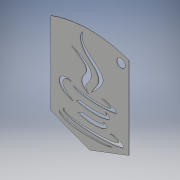
# Autodesk Inventor part: Деталь1
Saved by Autodesk Inventor 2018 (Build 220112000, 112)
## iProperties
Created: 2019-05-28
Part Number: Деталь1
Material: Типовые
Document SubType Name: Modeling
Designer: Vdalilsav
Density: 1 g/cm^3
Appearance: По умолчанию
Author: Vdalilsav
Autodesk Inventor part; units mm, degrees
ref_plane "YZ Plane" through (0, 0, 0) normal (1, 0, 0) x (0, 1, 0)
ref_plane "XZ Plane" through (0, 0, 0) normal (0, 1, 0) x (-1, 0, 0)
ref_plane "XY Plane" through (0, 0, 0) normal (0, 0, 1) x (1, 0, 0)
sketch "Эскиз1" plane through (0, 0, 0) normal (0, 1, 0) x (-1, 0, 0)
  line L0 (-168.2014, 197.6883) -> (149.2986, 197.6883) construction
  line L1 (149.2986, 197.6883) -> (149.2986, -384.3951) construction
  line L2 (149.2986, -384.3951) -> (-168.2014, -384.3951) construction
  line L3 (-168.2014, -384.3951) -> (-168.2014, 197.6883) construction
  line L4 (-172.8134, 183.0403) -> (-172.8134, -183.0403)
  line L5 (172.8134, -183.0403) -> (172.8134, 183.0403)
  line L6 (172.8134, 183.0403) -> (-172.8134, -183.0403) construction
  line L7 (-172.8134, 183.0403) -> (172.8134, -183.0403) construction
  line L8 (172.8134, -183.0403) -> (0, -248.8926)
  line L9 (-172.8134, -183.0403) -> (0, -248.8926)
  arc A0 (172.8134, 183.0403) -> (-172.8134, 183.0403) centre (0, -289.2463) ccw
  point P0 (0, 0)
  constraints: 12 end point, 2 midpoint, 2 point on circle, 1 centre point, 1 parallel, 2 other
sketch "Эскиз2" plane through (0, 0, 0) normal (0, 1, 0) x (-1, 0, 0)
  line L0 (-100.5732, -187.6969) -> (-90.8844, -191.9808) construction
  line L1 (-90.8844, -191.9808) -> (-75.4303, -195.3039) construction
  line L2 (-75.4303, -195.3039) -> (-57.8073, -197.5462) construction
  line L3 (-57.8073, -197.5462) -> (-50.4484, -198.1122) construction
  line L4 (-50.4484, -198.1122) -> (11.3731, -199.5671) construction
  line L5 (11.3731, -199.5671) -> (22.1637, -199.159) construction
  line L6 (22.1637, -199.159) -> (72.6522, -194.6635) construction
  line L7 (72.6522, -194.6635) -> (84.5907, -192.6655) construction
  line L8 (84.5907, -192.6655) -> (101.2161, -188.5411) construction
  line L9 (101.2161, -188.5411) -> (113.2372, -184.745) construction
  line L10 (113.2372, -184.745) -> (121.2017, -180.7255) construction
  line L11 (121.2017, -180.7255) -> (127.9007, -176.5944) construction
  line L12 (127.9007, -176.5944) -> (132.2272, -172.7909) construction
  line L13 (132.2272, -172.7909) -> (135.5715, -167.456) construction
  line L14 (135.5715, -167.456) -> (136.6862, -164.271) construction
  line L15 (136.6862, -164.271) -> (136.8189, -162.6519) construction
  line L16 (136.8189, -162.6519) -> (135.253, -164.271) construction
  line L17 (135.253, -164.271) -> (131.9353, -167.1375) construction
  line L18 (131.9353, -167.1375) -> (128.5645, -169.4201) construction
  line L19 (128.5645, -169.4201) -> (123.3836, -172.1896) construction
  line L20 (123.3836, -172.1896) -> (115.4536, -175.3114) construction
  line L21 (115.4536, -175.3114) -> (105.0835, -178.6485) construction
  line L22 (105.0835, -178.6485) -> (97.8352, -180.7655) construction
  line L23 (97.8352, -180.7655) -> (89.5822, -182.8826) construction
  line L24 (89.5822, -182.8826) -> (69.3615, -186.6907) construction
  line L25 (69.3615, -186.6907) -> (41.7588, -190.329) construction
  line L26 (41.7588, -190.329) -> (25.8958, -191.6874) construction
  line L27 (25.8958, -191.6874) -> (13.6226, -192.4635) construction
  line L28 (13.6226, -192.4635) -> (-0.2444, -193.1249) construction
  line L29 (-0.2444, -193.1249) -> (-15.9321, -193.513) construction
  line L30 (-15.9321, -193.513) -> (-21.243, -193.3904) construction
  line L31 (-21.243, -193.3904) -> (-33.8836, -193.3904) construction
  line L32 (-33.8836, -193.3904) -> (-40.4709, -193.2688) construction
  line L33 (-40.4709, -193.2688) -> (-51.2014, -192.7429) construction
  line L34 (-51.2014, -192.7429) -> (-59.6148, -192.1507) construction
  line L35 (-59.6148, -192.1507) -> (-65.0181, -191.7806) construction
  line L36 (-65.0181, -191.7806) -> (-74.3451, -191.0632) construction
  line L37 (-74.3451, -191.0632) -> (-76.1112, -190.9177) construction
  line L38 (-76.1112, -190.9177) -> (-91.5755, -189.204) construction
  line L39 (-91.5755, -189.204) -> (-94.5965, -188.6807) construction
  line L40 (-94.5965, -188.6807) -> (-97.0229, -188.3952) construction
  line L41 (-97.0229, -188.3952) -> (-98.5454, -188.1335) construction
  line L42 (-98.5454, -188.1335) -> (-100.5732, -187.6969) construction
  spline S0 degree 4 poles (-100.5732, -187.6969) (-90.8844, -191.9808) (-75.4303, -195.3039) (-57.8073, -197.5462) (-50.4484, -198.1122) (11.3731, -199.5671) (22.1637, -199.159) (72.6522, -194.6635) (84.5907, -192.6655) (101.2161, -188.5411) (113.2372, -184.745) (121.2017, -180.7255) (127.9007, -176.5944) (132.2272, -172.7909) (135.5715, -167.456) (136.6862, -164.271) (136.8189, -162.6519) (135.253, -164.271) (131.9353, -167.1375) (128.5645, -169.4201) (123.3836, -172.1896) (115.4536, -175.3114) (105.0835, -178.6485) (97.8352, -180.7655) (89.5822, -182.8826) (69.3615, -186.6907) (41.7588, -190.329) (25.8958, -191.6874) (13.6226, -192.4635) (-0.2444, -193.1249) (-15.9321, -193.513) (-21.243, -193.3904) (-33.8836, -193.3904) (-40.4709, -193.2688) (-51.2014, -192.7429) (-59.6148, -192.1507) (-65.0181, -191.7806) (-74.3451, -191.0632) (-76.1112, -190.9177) (-91.5755, -189.204) (-94.5965, -188.6807) (-97.0229, -188.3952) (-98.5454, -188.1335) (-100.5732, -187.6969) knots 1 1 1 1 1 2 3 4 5 6 7 8 9 10 11 12 13 14 15 16 17 18 19 20 21 22 23 24 25 26 27 28 29 30 31 32 33 34 35 36 37 38 39 40 41 41 41 41 41
  line L43 (111.9403, -142.3432) -> (113.6459, -144.4752) construction
  line L44 (113.6459, -144.4752) -> (114.6054, -147.6732) construction
  line L45 (114.6054, -147.6732) -> (113.7952, -150.1677) construction
  line L46 (113.7952, -150.1677) -> (110.892, -153.4059) construction
  line L47 (110.892, -153.4059) -> (108.3804, -154.9455) construction
  line L48 (108.3804, -154.9455) -> (102.2402, -157.513) construction
  line L49 (102.2402, -157.513) -> (97.2683, -159.1703) construction
  line L50 (97.2683, -159.1703) -> (86.7866, -161.5025) construction
  line L51 (86.7866, -161.5025) -> (78.9079, -162.7514) construction
  line L52 (78.9079, -162.7514) -> (72.2047, -164.0736) construction
  line L53 (72.2047, -164.0736) -> (49.1932, -166.8955) construction
  line L54 (49.1932, -166.8955) -> (37.3998, -167.7645) construction
  line L55 (37.3998, -167.7645) -> (18.7176, -169.2206) construction
  line L56 (18.7176, -169.2206) -> (-3.2892, -169.9456) construction
  line L57 (-3.2892, -169.9456) -> (-37.5273, -169.9456) construction
  line L58 (-37.5273, -169.9456) -> (-70.3936, -168.8122) construction
  line L59 (-70.3936, -168.8122) -> (-96.3775, -166.0991) construction
  line L60 (-96.3775, -166.0991) -> (-107.3306, -164.11) construction
  line L61 (-107.3306, -164.11) -> (-118.6934, -161.143) construction
  line L62 (-118.6934, -161.143) -> (-125.7296, -158.4458) construction
  line L63 (-125.7296, -158.4458) -> (-127.6116, -155.8998) construction
  line L64 (-127.6116, -155.8998) -> (-127.6116, -154.0071) construction
  line L65 (-127.6116, -154.0071) -> (-122.7322, -149.8816) construction
  line L66 (-122.7322, -149.8816) -> (-119.7589, -148.3776) construction
  line L67 (-119.7589, -148.3776) -> (-107.9616, -143.9347) construction
  line L68 (-107.9616, -143.9347) -> (-99.7456, -142.3432) construction
  line L69 (-99.7456, -142.3432) -> (-94.4887, -141.5856) construction
  line L70 (-94.4887, -141.5856) -> (-90.6183, -141.5856) construction
  line L71 (-90.6183, -141.5856) -> (-89.6238, -141.1555) construction
  line L72 (-89.6238, -141.1555) -> (-92.4191, -139.9192) construction
  line L73 (-92.4191, -139.9192) -> (-100.3212, -138.9516) construction
  line L74 (-100.3212, -138.9516) -> (-106.2881, -139.3547) construction
  line L75 (-106.2881, -139.3547) -> (-117.309, -141.3671) construction
  line L76 (-117.309, -141.3671) -> (-124.6465, -143.4482) construction
  line L77 (-124.6465, -143.4482) -> (-132.0085, -146.0648) construction
  line L78 (-132.0085, -146.0648) -> (-139.1832, -149.2139) construction
  line L79 (-139.1832, -149.2139) -> (-146.6729, -153.6575) construction
  line L80 (-146.6729, -153.6575) -> (-151.7202, -158.4964) construction
  line L81 (-151.7202, -158.4964) -> (-152.3684, -159.7625) construction
  line L82 (-152.3684, -159.7625) -> (-152.744, -162.9865) construction
  line L83 (-152.744, -162.9865) -> (-150.9599, -166.2105) construction
  line L84 (-150.9599, -166.2105) -> (-145.5761, -169.0589) construction
  line L85 (-145.5761, -169.0589) -> (-119.9974, -174.2608) construction
  line L86 (-119.9974, -174.2608) -> (-101.9283, -176.7574) construction
  line L87 (-101.9283, -176.7574) -> (-87.3291, -178.2385) construction
  line L88 (-87.3291, -178.2385) -> (-48.1035, -180.7168) construction
  line L89 (-48.1035, -180.7168) -> (-31.7211, -180.7168) construction
  line L90 (-31.7211, -180.7168) -> (22.8506, -178.8966) construction
  line L91 (22.8506, -178.8966) -> (35.2716, -177.6179) construction
  line L92 (35.2716, -177.6179) -> (61.13, -174.1701) construction
  line L93 (61.13, -174.1701) -> (82.266, -169.9038) construction
  line L94 (82.266, -169.9038) -> (93.8598, -166.6471) construction
  line L95 (93.8598, -166.6471) -> (105.7687, -161.9975) construction
  line L96 (105.7687, -161.9975) -> (113.4351, -158.2051) construction
  line L97 (113.4351, -158.2051) -> (118.7211, -153.0885) construction
  line L98 (118.7211, -153.0885) -> (119.8393, -149.2257) construction
  line L99 (119.8393, -149.2257) -> (118.6194, -146.8538) construction
  line L100 (118.6194, -146.8538) -> (116.4169, -144.8207) construction
  line L101 (116.4169, -144.8207) -> (112.6896, -142.6182) construction
  line L102 (112.6896, -142.6182) -> (111.9403, -142.3432) construction
  spline S1 degree 4 poles (111.9403, -142.3432) (113.6459, -144.4752) (114.6054, -147.6732) (113.7952, -150.1677) (110.892, -153.4059) (108.3804, -154.9455) (102.2402, -157.513) (97.2683, -159.1703) (86.7866, -161.5025) (78.9079, -162.7514) (72.2047, -164.0736) (49.1932, -166.8955) (37.3998, -167.7645) (18.7176, -169.2206) (-3.2892, -169.9456) (-37.5273, -169.9456) (-70.3936, -168.8122) (-96.3775, -166.0991) (-107.3306, -164.11) (-118.6934, -161.143) (-125.7296, -158.4458) (-127.6116, -155.8998) (-127.6116, -154.0071) (-122.7322, -149.8816) (-119.7589, -148.3776) (-107.9616, -143.9347) (-99.7456, -142.3432) (-94.4887, -141.5856) (-90.6183, -141.5856) (-89.6238, -141.1555) (-92.4191, -139.9192) (-100.3212, -138.9516) (-106.2881, -139.3547) (-117.309, -141.3671) (-124.6465, -143.4482) (-132.0085, -146.0648) (-139.1832, -149.2139) (-146.6729, -153.6575) (-151.7202, -158.4964) (-152.3684, -159.7625) (-152.744, -162.9865) (-150.9599, -166.2105) (-145.5761, -169.0589) (-119.9974, -174.2608) (-101.9283, -176.7574) (-87.3291, -178.2385) (-48.1035, -180.7168) (-31.7211, -180.7168) (22.8506, -178.8966) (35.2716, -177.6179) (61.13, -174.1701) (82.266, -169.9038) (93.8598, -166.6471) (105.7687, -161.9975) (113.4351, -158.2051) (118.7211, -153.0885) (119.8393, -149.2257) (118.6194, -146.8538) (116.4169, -144.8207) (112.6896, -142.6182) (111.9403, -142.3432) knots 1 1 1 1 1 2 3 4 5 6 7 8 9 10 11 12 13 14 15 16 17 18 19 20 21 22 23 24 25 26 27 28 29 30 31 32 33 34 35 36 37 38 39 40 41 42 43 44 45 46 47 48 49 50 51 52 53 54 55 56 57 58 58 58 58 58
  line L103 (53.8313, -129.4967) -> (45.6691, -125.709) construction
  line L104 (45.6691, -125.709) -> (37.8803, -121.7613) construction
  line L105 (37.8803, -121.7613) -> (32.919, -118.8805) construction
  line L106 (32.919, -118.8805) -> (31.7453, -118.8805) construction
  line L107 (31.7453, -118.8805) -> (24.0099, -120.5343) construction
  line L108 (24.0099, -120.5343) -> (10.833, -122.4014) construction
  line L109 (10.833, -122.4014) -> (-3.0465, -123.9641) construction
  line L110 (-3.0465, -123.9641) -> (-13.6498, -124.4325) construction
  line L111 (-13.6498, -124.4325) -> (-29.6187, -124.0493) construction
  line L112 (-29.6187, -124.0493) -> (-45.0884, -122.4699) construction
  line L113 (-45.0884, -122.4699) -> (-54.8927, -121.3305) construction
  line L114 (-54.8927, -121.3305) -> (-60.8755, -119.3267) construction
  line L115 (-60.8755, -119.3267) -> (-63.781, -116.7933) construction
  line L116 (-63.781, -116.7933) -> (-63.781, -115.1902) construction
  line L117 (-63.781, -115.1902) -> (-63.1701, -113.4782) construction
  line L118 (-63.1701, -113.4782) -> (-61.1647, -112.0951) construction
  line L119 (-61.1647, -112.0951) -> (-59.7643, -110.8331) construction
  line L120 (-59.7643, -110.8331) -> (-61.9599, -111.0406) construction
  line L121 (-61.9599, -111.0406) -> (-64.7087, -112.0606) construction
  line L122 (-64.7087, -112.0606) -> (-67.5785, -113.167) construction
  line L123 (-67.5785, -113.167) -> (-71.2609, -114.9131) construction
  line L124 (-71.2609, -114.9131) -> (-73.5762, -116.2658) construction
  line L125 (-73.5762, -116.2658) -> (-75.7428, -118.1564) construction
  line L126 (-75.7428, -118.1564) -> (-77.9326, -120.7925) construction
  line L127 (-77.9326, -120.7925) -> (-78.3711, -123.2774) construction
  line L128 (-78.3711, -123.2774) -> (-76.3092, -128.1495) construction
  line L129 (-76.3092, -128.1495) -> (-73.0589, -130.8664) construction
  line L130 (-73.0589, -130.8664) -> (-63.8418, -135.664) construction
  line L131 (-63.8418, -135.664) -> (-50.1798, -139.754) construction
  line L132 (-50.1798, -139.754) -> (-38.7359, -141.6675) construction
  line L133 (-38.7359, -141.6675) -> (-23.6859, -143.0657) construction
  line L134 (-23.6859, -143.0657) -> (-0.2774, -142.5492) construction
  line L135 (-0.2774, -142.5492) -> (14.7613, -140.7575) construction
  line L136 (14.7613, -140.7575) -> (32.8343, -136.8467) construction
  line L137 (32.8343, -136.8467) -> (45.768, -132.9355) construction
  line L138 (45.768, -132.9355) -> (51.2349, -130.6243) construction
  line L139 (51.2349, -130.6243) -> (53.8313, -129.4967) construction
  spline S2 degree 4 poles (53.8313, -129.4967) (45.6691, -125.709) (37.8803, -121.7613) (32.919, -118.8805) (31.7453, -118.8805) (24.0099, -120.5343) (10.833, -122.4014) (-3.0465, -123.9641) (-13.6498, -124.4325) (-29.6187, -124.0493) (-45.0884, -122.4699) (-54.8927, -121.3305) (-60.8755, -119.3267) (-63.781, -116.7933) (-63.781, -115.1902) (-63.1701, -113.4782) (-61.1647, -112.0951) (-59.7643, -110.8331) (-61.9599, -111.0406) (-64.7087, -112.0606) (-67.5785, -113.167) (-71.2609, -114.9131) (-73.5762, -116.2658) (-75.7428, -118.1564) (-77.9326, -120.7925) (-78.3711, -123.2774) (-76.3092, -128.1495) (-73.0589, -130.8664) (-63.8418, -135.664) (-50.1798, -139.754) (-38.7359, -141.6675) (-23.6859, -143.0657) (-0.2774, -142.5492) (14.7613, -140.7575) (32.8343, -136.8467) (45.768, -132.9355) (51.2349, -130.6243) (53.8313, -129.4967) knots 1 1 1 1 1 2 3 4 5 6 7 8 9 10 11 12 13 14 15 16 17 18 19 20 21 22 23 24 25 26 27 28 29 30 31 32 33 34 35 35 35 35 35
  line L140 (74.2215, -96.4018) -> (75.9291, -94.3283) construction
  line L141 (75.9291, -94.3283) -> (82.857, -90.6692) construction
  line L142 (82.857, -90.6692) -> (97.9787, -80.6075) construction
  line L143 (97.9787, -80.6075) -> (105.2012, -74.7702) construction
  line L144 (105.2012, -74.7702) -> (109.8782, -70.0928) construction
  line L145 (109.8782, -70.0928) -> (114.347, -64.354) construction
  line L146 (114.347, -64.354) -> (117.6643, -58.7901) construction
  line L147 (117.6643, -58.7901) -> (119.2836, -54.614) construction
  line L148 (119.2836, -54.614) -> (120.4768, -49.9834) construction
  line L149 (120.4768, -49.9834) -> (119.9848, -41.7758) construction
  line L150 (119.9848, -41.7758) -> (118.7174, -38.3192) construction
  line L151 (118.7174, -38.3192) -> (116.6819, -34.4018) construction
  line L152 (116.6819, -34.4018) -> (113.4558, -30.9836) construction
  line L153 (113.4558, -30.9836) -> (109.6919, -28.2183) construction
  line L154 (109.6919, -28.2183) -> (104.5675, -25.5263) construction
  line L155 (104.5675, -25.5263) -> (99.7968, -24.5399) construction
  line L156 (99.7968, -24.5399) -> (96.0287, -24.1356) construction
  line L157 (96.0287, -24.1356) -> (90.9669, -24.5075) construction
  line L158 (90.9669, -24.5075) -> (86.3903, -25.8336) construction
  line L159 (86.3903, -25.8336) -> (83.5148, -26.9478) construction
  line L160 (83.5148, -26.9478) -> (82.9984, -26.5089) construction
  line L161 (82.9984, -26.5089) -> (83.8891, -25.6311) construction
  line L162 (83.8891, -25.6311) -> (86.4193, -23.6044) construction
  line L163 (86.4193, -23.6044) -> (95.0019, -20.0576) construction
  line L164 (95.0019, -20.0576) -> (104.5184, -19.0207) construction
  line L165 (104.5184, -19.0207) -> (113.4425, -20.1316) construction
  line L166 (113.4425, -20.1316) -> (118.5526, -22.0201) construction
  line L167 (118.5526, -22.0201) -> (125.0919, -25.4171) construction
  line L168 (125.0919, -25.4171) -> (131.1994, -30.7962) construction
  line L169 (131.1994, -30.7962) -> (134.5053, -36.1752) construction
  line L170 (134.5053, -36.1752) -> (136.4104, -42.1707) construction
  line L171 (136.4104, -42.1707) -> (136.4104, -50.5755) construction
  line L172 (136.4104, -50.5755) -> (133.1038, -60.7047) construction
  line L173 (133.1038, -60.7047) -> (128.5343, -67.1201) construction
  line L174 (128.5343, -67.1201) -> (115.5534, -79.2307) construction
  line L175 (115.5534, -79.2307) -> (109.5119, -82.736) construction
  line L176 (109.5119, -82.736) -> (93.882, -90.2067) construction
  line L177 (93.882, -90.2067) -> (79.4154, -95.2427) construction
  line L178 (79.4154, -95.2427) -> (74.9257, -96.5594) construction
  line L179 (74.9257, -96.5594) -> (74.2215, -96.4018) construction
  spline S3 degree 4 poles (74.2215, -96.4018) (75.9291, -94.3283) (82.857, -90.6692) (97.9787, -80.6075) (105.2012, -74.7702) (109.8782, -70.0928) (114.347, -64.354) (117.6643, -58.7901) (119.2836, -54.614) (120.4768, -49.9834) (119.9848, -41.7758) (118.7174, -38.3192) (116.6819, -34.4018) (113.4558, -30.9836) (109.6919, -28.2183) (104.5675, -25.5263) (99.7968, -24.5399) (96.0287, -24.1356) (90.9669, -24.5075) (86.3903, -25.8336) (83.5148, -26.9478) (82.9984, -26.5089) (83.8891, -25.6311) (86.4193, -23.6044) (95.0019, -20.0576) (104.5184, -19.0207) (113.4425, -20.1316) (118.5526, -22.0201) (125.0919, -25.4171) (131.1994, -30.7962) (134.5053, -36.1752) (136.4104, -42.1707) (136.4104, -50.5755) (133.1038, -60.7047) (128.5343, -67.1201) (115.5534, -79.2307) (109.5119, -82.736) (93.882, -90.2067) (79.4154, -95.2427) (74.9257, -96.5594) (74.2215, -96.4018) knots 1 1 1 1 1 2 3 4 5 6 7 8 9 10 11 12 13 14 15 16 17 18 19 20 21 22 23 24 25 26 27 28 29 30 31 32 33 34 35 36 37 38 38 38 38 38
  line L180 (60.7679, -87.5507) -> (57.2554, -85.8918) construction
  line L181 (57.2554, -85.8918) -> (54.6702, -84.5782) construction
  line L182 (54.6702, -84.5782) -> (48.1108, -80.561) construction
  line L183 (48.1108, -80.561) -> (45.9948, -78.3884) construction
  line L184 (45.9948, -78.3884) -> (45.258, -77.5949) construction
  line L185 (45.258, -77.5949) -> (32.9691, -79.621) construction
  line L186 (32.9691, -79.621) -> (15.1394, -82.6017) construction
  line L187 (15.1394, -82.6017) -> (0.3446, -83.9023) construction
  line L188 (0.3446, -83.9023) -> (-15.9332, -84.9251) construction
  line L189 (-15.9332, -84.9251) -> (-33.9822, -84.5386) construction
  line L190 (-33.9822, -84.5386) -> (-44.6106, -83.8816) construction
  line L191 (-44.6106, -83.8816) -> (-62.0188, -82.5002) construction
  line L192 (-62.0188, -82.5002) -> (-68.374, -81.2971) construction
  line L193 (-68.374, -81.2971) -> (-72.2303, -79.3535) construction
  line L194 (-72.2303, -79.3535) -> (-74.4515, -76.2376) construction
  line L195 (-74.4515, -76.2376) -> (-73.4643, -72.443) construction
  line L196 (-73.4643, -72.443) -> (-71.2739, -69.7282) construction
  line L197 (-71.2739, -69.7282) -> (-69.392, -68.3707) construction
  line L198 (-69.392, -68.3707) -> (-69.1144, -67.4144) construction
  line L199 (-69.1144, -67.4144) -> (-70.8729, -67.7537) construction
  line L200 (-70.8729, -67.7537) -> (-72.8164, -69.0495) construction
  line L201 (-72.8164, -69.0495) -> (-76.1174, -70.3452) construction
  line L202 (-76.1174, -70.3452) -> (-80.6524, -72.3505) construction
  line L203 (-80.6524, -72.3505) -> (-84.4406, -74.4358) construction
  line L204 (-84.4406, -74.4358) -> (-88.8044, -77.974) construction
  line L205 (-88.8044, -77.974) -> (-89.7086, -80.4704) construction
  line L206 (-89.7086, -80.4704) -> (-89.5907, -83.989) construction
  line L207 (-89.5907, -83.989) -> (-85.8534, -88.4964) construction
  line L208 (-85.8534, -88.4964) -> (-80.2462, -91.4196) construction
  line L209 (-80.2462, -91.4196) -> (-71.8486, -94.396) construction
  line L210 (-71.8486, -94.396) -> (-63.0258, -96.2296) construction
  line L211 (-63.0258, -96.2296) -> (-50.3691, -98.0763) construction
  line L212 (-50.3691, -98.0763) -> (-29.095, -99.5334) construction
  line L213 (-29.095, -99.5334) -> (-3.4781, -98.866) construction
  line L214 (-3.4781, -98.866) -> (25.7568, -95.4316) construction
  line L215 (25.7568, -95.4316) -> (44.6538, -91.8335) construction
  line L216 (44.6538, -91.8335) -> (59.4549, -88.2376) construction
  line L217 (59.4549, -88.2376) -> (60.7679, -87.5507) construction
  spline S4 degree 4 poles (60.7679, -87.5507) (57.2554, -85.8918) (54.6702, -84.5782) (48.1108, -80.561) (45.9948, -78.3884) (45.258, -77.5949) (32.9691, -79.621) (15.1394, -82.6017) (0.3446, -83.9023) (-15.9332, -84.9251) (-33.9822, -84.5386) (-44.6106, -83.8816) (-62.0188, -82.5002) (-68.374, -81.2971) (-72.2303, -79.3535) (-74.4515, -76.2376) (-73.4643, -72.443) (-71.2739, -69.7282) (-69.392, -68.3707) (-69.1144, -67.4144) (-70.8729, -67.7537) (-72.8164, -69.0495) (-76.1174, -70.3452) (-80.6524, -72.3505) (-84.4406, -74.4358) (-88.8044, -77.974) (-89.7086, -80.4704) (-89.5907, -83.989) (-85.8534, -88.4964) (-80.2462, -91.4196) (-71.8486, -94.396) (-63.0258, -96.2296) (-50.3691, -98.0763) (-29.095, -99.5334) (-3.4781, -98.866) (25.7568, -95.4316) (44.6538, -91.8335) (59.4549, -88.2376) (60.7679, -87.5507) knots 1 1 1 1 1 2 3 4 5 6 7 8 9 10 11 12 13 14 15 16 17 18 19 20 21 22 23 24 25 26 27 28 29 30 31 32 33 34 35 36 36 36 36 36
  line L218 (75.5916, -37.4918) -> (68.9093, -40.7755) construction
  line L219 (68.9093, -40.7755) -> (62.135, -44.3349) construction
  line L220 (62.135, -44.3349) -> (58.7594, -46.5624) construction
  line L221 (58.7594, -46.5624) -> (54.1673, -48.0342) construction
  line L222 (54.1673, -48.0342) -> (28.0322, -52.8418) construction
  line L223 (28.0322, -52.8418) -> (15.273, -54.4786) construction
  line L224 (15.273, -54.4786) -> (-12.7561, -56.6644) construction
  line L225 (-12.7561, -56.6644) -> (-33.4668, -57.3453) construction
  line L226 (-33.4668, -57.3453) -> (-71.0949, -56.7546) construction
  line L227 (-71.0949, -56.7546) -> (-80.2109, -56.1071) construction
  line L228 (-80.2109, -56.1071) -> (-107.865, -52.1466) construction
  line L229 (-107.865, -52.1466) -> (-114.7802, -50.0062) construction
  line L230 (-114.7802, -50.0062) -> (-118.4399, -48.2008) construction
  line L231 (-118.4399, -48.2008) -> (-120.5943, -46.1797) construction
  line L232 (-120.5943, -46.1797) -> (-121.4605, -44.0697) construction
  line L233 (-121.4605, -44.0697) -> (-120.5679, -42.0263) construction
  line L234 (-120.5679, -42.0263) -> (-116.6144, -39.172) construction
  line L235 (-116.6144, -39.172) -> (-110.2588, -35.7407) construction
  line L236 (-110.2588, -35.7407) -> (-99.4189, -31.4398) construction
  line L237 (-99.4189, -31.4398) -> (-88.5091, -27.8381) construction
  line L238 (-88.5091, -27.8381) -> (-79.379, -25.5987) construction
  line L239 (-79.379, -25.5987) -> (-68.1026, -23.5612) construction
  line L240 (-68.1026, -23.5612) -> (-60.1477, -23.0308) construction
  line L241 (-60.1477, -23.0308) -> (-52.7568, -23.0308) construction
  line L242 (-52.7568, -23.0308) -> (-54.0936, -23.7675) construction
  line L243 (-54.0936, -23.7675) -> (-57.6807, -24.5473) construction
  line L244 (-57.6807, -24.5473) -> (-63.3621, -25.9955) construction
  line L245 (-63.3621, -25.9955) -> (-69.6005, -27.9561) construction
  line L246 (-69.6005, -27.9561) -> (-75.3264, -29.8722) construction
  line L247 (-75.3264, -29.8722) -> (-81.542, -32.0756) construction
  line L248 (-81.542, -32.0756) -> (-86.1304, -34.1741) construction
  line L249 (-86.1304, -34.1741) -> (-91.0667, -37.1972) construction
  line L250 (-91.0667, -37.1972) -> (-92.6007, -38.6774) construction
  line L251 (-92.6007, -38.6774) -> (-92.9505, -40.2113) construction
  line L252 (-92.9505, -40.2113) -> (-91.3897, -42.3104) construction
  line L253 (-91.3897, -42.3104) -> (-88.268, -44.0058) construction
  line L254 (-88.268, -44.0058) -> (-78.7023, -46.0417) construction
  line L255 (-78.7023, -46.0417) -> (-67.9187, -47.0942) construction
  line L256 (-67.9187, -47.0942) -> (-57.1782, -47.6957) construction
  line L257 (-57.1782, -47.6957) -> (-15.8045, -47.121) construction
  line L258 (-15.8045, -47.121) -> (-3.9267, -46.5112) construction
  line L259 (-3.9267, -46.5112) -> (35.5406, -43.5463) construction
  line L260 (35.5406, -43.5463) -> (49.9103, -41.3869) construction
  line L261 (49.9103, -41.3869) -> (56.3099, -40.5624) construction
  line L262 (56.3099, -40.5624) -> (70.9693, -38.4615) construction
  line L263 (70.9693, -38.4615) -> (75.5916, -37.4918) construction
  spline S5 degree 4 poles (75.5916, -37.4918) (68.9093, -40.7755) (62.135, -44.3349) (58.7594, -46.5624) (54.1673, -48.0342) (28.0322, -52.8418) (15.273, -54.4786) (-12.7561, -56.6644) (-33.4668, -57.3453) (-71.0949, -56.7546) (-80.2109, -56.1071) (-107.865, -52.1466) (-114.7802, -50.0062) (-118.4399, -48.2008) (-120.5943, -46.1797) (-121.4605, -44.0697) (-120.5679, -42.0263) (-116.6144, -39.172) (-110.2588, -35.7407) (-99.4189, -31.4398) (-88.5091, -27.8381) (-79.379, -25.5987) (-68.1026, -23.5612) (-60.1477, -23.0308) (-52.7568, -23.0308) (-54.0936, -23.7675) (-57.6807, -24.5473) (-63.3621, -25.9955) (-69.6005, -27.9561) (-75.3264, -29.8722) (-81.542, -32.0756) (-86.1304, -34.1741) (-91.0667, -37.1972) (-92.6007, -38.6774) (-92.9505, -40.2113) (-91.3897, -42.3104) (-88.268, -44.0058) (-78.7023, -46.0417) (-67.9187, -47.0942) (-57.1782, -47.6957) (-15.8045, -47.121) (-3.9267, -46.5112) (35.5406, -43.5463) (49.9103, -41.3869) (56.3099, -40.5624) (70.9693, -38.4615) (75.5916, -37.4918) knots 1 1 1 1 1 2 3 4 5 6 7 8 9 10 11 12 13 14 15 16 17 18 19 20 21 22 23 24 25 26 27 28 29 30 31 32 33 34 35 36 37 38 39 40 41 42 43 44 44 44 44 44
  line L264 (31.4979, 192.7775) -> (34.3008, 189.3991) construction
  line L265 (34.3008, 189.3991) -> (37.2522, 184.3131) construction
  line L266 (37.2522, 184.3131) -> (40.2072, 176.4998) construction
  line L267 (40.2072, 176.4998) -> (41.7543, 168.6302) construction
  line L268 (41.7543, 168.6302) -> (41.7543, 159.3919) construction
  line L269 (41.7543, 159.3919) -> (40.4358, 151.7232) construction
  line L270 (40.4358, 151.7232) -> (38.7384, 146.146) construction
  line L271 (38.7384, 146.146) -> (33.9109, 135.2699) construction
  line L272 (33.9109, 135.2699) -> (29.6542, 127.4494) construction
  line L273 (29.6542, 127.4494) -> (23.1207, 118.6886) construction
  line L274 (23.1207, 118.6886) -> (17.0821, 111.8086) construction
  line L275 (17.0821, 111.8086) -> (3.2217, 98.3842) construction
  line L276 (3.2217, 98.3842) -> (-7.0856, 89.5595) construction
  line L277 (-7.0856, 89.5595) -> (-21.124, 77.4552) construction
  line L278 (-21.124, 77.4552) -> (-28.1746, 69.176) construction
  line L279 (-28.1746, 69.176) -> (-33.0887, 61.9652) construction
  line L280 (-33.0887, 61.9652) -> (-38.3234, 49.6071) construction
  line L281 (-38.3234, 49.6071) -> (-39.0482, 41.6768) construction
  line L282 (-39.0482, 41.6768) -> (-39.0482, 36.4647) construction
  line L283 (-39.0482, 36.4647) -> (-38.0674, 30.7483) construction
  line L284 (-38.0674, 30.7483) -> (-36.2431, 25.0319) construction
  line L285 (-36.2431, 25.0319) -> (-33.5977, 19.8932) construction
  line L286 (-33.5977, 19.8932) -> (-27.6244, 9.2545) construction
  line L287 (-27.6244, 9.2545) -> (-19.7015, -1.6857) construction
  line L288 (-19.7015, -1.6857) -> (-16.8001, -6.1297) construction
  line L289 (-16.8001, -6.1297) -> (-10.2962, -16.7856) construction
  line L290 (-10.2962, -16.7856) -> (-7.1654, -22.293) construction
  line L291 (-7.1654, -22.293) -> (-8.2431, -21.9752) construction
  line L292 (-8.2431, -21.9752) -> (-9.7906, -20.3863) construction
  line L293 (-9.7906, -20.3863) -> (-16.9077, -14.0378) construction
  line L294 (-16.9077, -14.0378) -> (-21.5394, -9.339) construction
  line L295 (-21.5394, -9.339) -> (-26.5068, -4.5059) construction
  line L296 (-26.5068, -4.5059) -> (-39.6694, 9.7173) construction
  line L297 (-39.6694, 9.7173) -> (-49.3175, 22.185) construction
  line L298 (-49.3175, 22.185) -> (-56.4992, 34.52) construction
  line L299 (-56.4992, 34.52) -> (-58.2724, 40.2107) construction
  line L300 (-58.2724, 40.2107) -> (-59.5095, 47.0973) construction
  line L301 (-59.5095, 47.0973) -> (-59.2621, 55.9633) construction
  line L302 (-59.2621, 55.9633) -> (-55.1937, 66.0399) construction
  line L303 (-55.1937, 66.0399) -> (-45.4468, 79.0724) construction
  line L304 (-45.4468, 79.0724) -> (-22.8039, 98.9706) construction
  line L305 (-22.8039, 98.9706) -> (-0.8324, 116.4489) construction
  line L306 (-0.8324, 116.4489) -> (13.3053, 130.0793) construction
  line L307 (13.3053, 130.0793) -> (19.392, 136.5912) construction
  line L308 (19.392, 136.5912) -> (24.4137, 143.7595) construction
  line L309 (24.4137, 143.7595) -> (29.972, 154.1861) construction
  line L310 (29.972, 154.1861) -> (31.812, 161.1627) construction
  line L311 (31.812, 161.1627) -> (33.7381, 171.4279) construction
  line L312 (33.7381, 171.4279) -> (33.3346, 175.3502) construction
  line L313 (33.3346, 175.3502) -> (32.6111, 186.948) construction
  line L314 (32.6111, 186.948) -> (31.6073, 191.7706) construction
  line L315 (31.6073, 191.7706) -> (31.4979, 192.7775) construction
  spline S6 degree 4 poles (31.4979, 192.7775) (34.3008, 189.3991) (37.2522, 184.3131) (40.2072, 176.4998) (41.7543, 168.6302) (41.7543, 159.3919) (40.4358, 151.7232) (38.7384, 146.146) (33.9109, 135.2699) (29.6542, 127.4494) (23.1207, 118.6886) (17.0821, 111.8086) (3.2217, 98.3842) (-7.0856, 89.5595) (-21.124, 77.4552) (-28.1746, 69.176) (-33.0887, 61.9652) (-38.3234, 49.6071) (-39.0482, 41.6768) (-39.0482, 36.4647) (-38.0674, 30.7483) (-36.2431, 25.0319) (-33.5977, 19.8932) (-27.6244, 9.2545) (-19.7015, -1.6857) (-16.8001, -6.1297) (-10.2962, -16.7856) (-7.1654, -22.293) (-8.2431, -21.9752) (-9.7906, -20.3863) (-16.9077, -14.0378) (-21.5394, -9.339) (-26.5068, -4.5059) (-39.6694, 9.7173) (-49.3175, 22.185) (-56.4992, 34.52) (-58.2724, 40.2107) (-59.5095, 47.0973) (-59.2621, 55.9633) (-55.1937, 66.0399) (-45.4468, 79.0724) (-22.8039, 98.9706) (-0.8324, 116.4489) (13.3053, 130.0793) (19.392, 136.5912) (24.4137, 143.7595) (29.972, 154.1861) (31.812, 161.1627) (33.7381, 171.4279) (33.3346, 175.3502) (32.6111, 186.948) (31.6073, 191.7706) (31.4979, 192.7775) knots 1 1 1 1 1 2 3 4 5 6 7 8 9 10 11 12 13 14 15 16 17 18 19 20 21 22 23 24 25 26 27 28 29 30 31 32 33 34 35 36 37 38 39 40 41 42 43 44 45 46 47 48 49 50 50 50 50 50
  line L316 (80.1358, 112.6955) -> (73.4162, 108.7122) construction
  line L317 (73.4162, 108.7122) -> (59.27, 99.9109) construction
  line L318 (59.27, 99.9109) -> (49.1445, 93.3154) construction
  line L319 (49.1445, 93.3154) -> (36.0562, 83.4339) construction
  line L320 (36.0562, 83.4339) -> (27.6772, 75.6481) construction
  line L321 (27.6772, 75.6481) -> (22.7748, 70.6541) construction
  line L322 (22.7748, 70.6541) -> (17.4117, 62.7347) construction
  line L323 (17.4117, 62.7347) -> (15.507, 57.3214) construction
  line L324 (15.507, 57.3214) -> (14.7551, 50.254) construction
  line L325 (14.7551, 50.254) -> (16.5596, 42.6855) construction
  line L326 (16.5596, 42.6855) -> (20.326, 35.595) construction
  line L327 (20.326, 35.595) -> (26.8875, 26.6729) construction
  line L328 (26.8875, 26.6729) -> (33.7043, 16.0049) construction
  line L329 (33.7043, 16.0049) -> (36.6503, 8.6752) construction
  line L330 (36.6503, 8.6752) -> (36.9514, -1.7811) construction
  line L331 (36.9514, -1.7811) -> (35.7023, -5.4011) construction
  line L332 (35.7023, -5.4011) -> (33.4629, -10.2806) construction
  line L333 (33.4629, -10.2806) -> (28.121, -18.2074) construction
  line L334 (28.121, -18.2074) -> (22.7445, -23.7562) construction
  line L335 (22.7445, -23.7562) -> (18.5191, -27.2977) construction
  line L336 (18.5191, -27.2977) -> (11.8434, -32.2386) construction
  line L337 (11.8434, -32.2386) -> (7.6053, -34.9616) construction
  line L338 (7.6053, -34.9616) -> (5.4532, -36.3889) construction
  line L339 (5.4532, -36.3889) -> (6.3975, -34.8518) construction
  line L340 (6.3975, -34.8518) -> (10.2623, -30.7454) construction
  line L341 (10.2623, -30.7454) -> (13.9296, -25.1018) construction
  line L342 (13.9296, -25.1018) -> (16.2422, -20.2757) construction
  line L343 (16.2422, -20.2757) -> (17.4092, -14.3873) construction
  line L344 (17.4092, -14.3873) -> (17.2501, -10.117) construction
  line L345 (17.2501, -10.117) -> (16.4704, -5.3847) construction
  line L346 (16.4704, -5.3847) -> (14.1396, 0.7112) construction
  line L347 (14.1396, 0.7112) -> (10.9482, 4.5839) construction
  line L348 (10.9482, 4.5839) -> (7.7209, 8.1698) construction
  line L349 (7.7209, 8.1698) -> (5.7845, 10.895) construction
  line L350 (5.7845, 10.895) -> (1.4707, 17.0605) construction
  line L351 (1.4707, 17.0605) -> (-1.8959, 23.2907) construction
  line L352 (-1.8959, 23.2907) -> (-4.6434, 29.7143) construction
  line L353 (-4.6434, 29.7143) -> (-6.5512, 36.1123) construction
  line L354 (-6.5512, 36.1123) -> (-7.0146, 41.2089) construction
  line L355 (-7.0146, 41.2089) -> (-6.1918, 51.9986) construction
  line L356 (-6.1918, 51.9986) -> (-3.7508, 59.1242) construction
  line L357 (-3.7508, 59.1242) -> (-0.8384, 64.727) construction
  line L358 (-0.8384, 64.727) -> (3.3993, 70.9869) construction
  line L359 (3.3993, 70.9869) -> (11.4331, 79.2782) construction
  line L360 (11.4331, 79.2782) -> (19.8504, 86.1128) construction
  line L361 (19.8504, 86.1128) -> (30.2462, 92.6596) construction
  line L362 (30.2462, 92.6596) -> (42.1168, 98.7388) construction
  line L363 (42.1168, 98.7388) -> (59.3691, 106.2383) construction
  line L364 (59.3691, 106.2383) -> (79.459, 112.6955) construction
  line L365 (79.459, 112.6955) -> (80.1358, 112.6955) construction
  spline S7 degree 4 poles (80.1358, 112.6955) (73.4162, 108.7122) (59.27, 99.9109) (49.1445, 93.3154) (36.0562, 83.4339) (27.6772, 75.6481) (22.7748, 70.6541) (17.4117, 62.7347) (15.507, 57.3214) (14.7551, 50.254) (16.5596, 42.6855) (20.326, 35.595) (26.8875, 26.6729) (33.7043, 16.0049) (36.6503, 8.6752) (36.9514, -1.7811) (35.7023, -5.4011) (33.4629, -10.2806) (28.121, -18.2074) (22.7445, -23.7562) (18.5191, -27.2977) (11.8434, -32.2386) (7.6053, -34.9616) (5.4532, -36.3889) (6.3975, -34.8518) (10.2623, -30.7454) (13.9296, -25.1018) (16.2422, -20.2757) (17.4092, -14.3873) (17.2501, -10.117) (16.4704, -5.3847) (14.1396, 0.7112) (10.9482, 4.5839) (7.7209, 8.1698) (5.7845, 10.895) (1.4707, 17.0605) (-1.8959, 23.2907) (-4.6434, 29.7143) (-6.5512, 36.1123) (-7.0146, 41.2089) (-6.1918, 51.9986) (-3.7508, 59.1242) (-0.8384, 64.727) (3.3993, 70.9869) (11.4331, 79.2782) (19.8504, 86.1128) (30.2462, 92.6596) (42.1168, 98.7388) (59.3691, 106.2383) (79.459, 112.6955) (80.1358, 112.6955) knots 1 1 1 1 1 2 3 4 5 6 7 8 9 10 11 12 13 14 15 16 17 18 19 20 21 22 23 24 25 26 27 28 29 30 31 32 33 34 35 36 37 38 39 40 41 42 43 44 45 46 47 48 48 48 48 48
  point P0 (0, 0)
  constraints: 7 horizontal, 5 vertical, 11 other
extrude "Выдавливание1" add sketch "Эскиз1" against normal blind 2
sketch "Эскиз3" plane through (0, 0, 0) normal (0, 1, 0) x (1, 0, 0)
  circle A0 centre (139.154, -156.1017) radius 18.8989
  point P0 (0, 0)
  constraints: 1 centre point
extrude "Выдавливание2" cut sketch "Эскиз3" against normal blind 2
extrude "Выдавливание3" cut sketch "Эскиз2" against normal blind 2
sketch "Эскиз4" plane through (0, 0, 0) normal (0, 1, 0) x (1, 0, 0)
  point P0 (0, 0)
